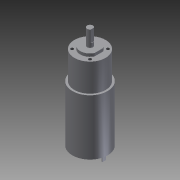
# Autodesk Inventor part: IG32P-Motor
Saved by Autodesk Inventor 2012 (Build 160160000, 160)
## iProperties
Created: 2013-07-13
Part Number: IG32P-Motor
Material: Default
Document SubType Name: Modeling
Designer: joe_000
Density: 2.67636 g/cm^3
Mass: 220 g
Surface Area: 122.703 cm^2
Volume: 82.2012 cm^3
Author: joe_000
Autodesk Inventor part; units mm, degrees
ref_plane "YZ Plane" through (0, 0, 0) normal (1, 0, 0) x (0, 1, 0)
ref_plane "XZ Plane" through (0, 0, 0) normal (0, 1, 0) x (-1, 0, 0)
ref_plane "XY Plane" through (0, 0, 0) normal (0, 0, 1) x (1, 0, 0)
sketch "Sketch1" plane through (0, 0, 0) normal (0, 0, 1) x (1, 0, 0)
  circle A0 centre (0, 0) radius 18
  dimension "d0" = 36
  constraints: 1 centre point, 1 coincident
  measures "d0" diameter of A0
extrude "Extrusion1" add sketch "Sketch1" along normal blind 57.1
sketch "Sketch2" plane through (0, 0, 57.1) normal (0, 0, 1) x (1, 0, 0)
  circle A0 centre (0, 0) radius 16
  dimension "d3" = 32
  constraints: 1 centre point
  measures "d3" diameter of A0
extrude "Extrusion2" add sketch "Sketch2" along normal blind 28.5
sketch "Sketch3" plane through (0, 0, 85.6) normal (0, 0, 1) x (1, 0, 0)
  line L0 (-9, 4.3589) -> (-9, -4.3589)
  line L1 (9, 4.3589) -> (9, -4.3589)
  arc A0 (9, 4.3589) -> (-9, 4.3589) centre (0, 0) ccw
  arc A1 (-9, -4.3589) -> (9, -4.3589) centre (0, 0) ccw
  circle A2 centre (0, 0) radius 16 projected
  dimension "d7" = 18
  dimension "d8" = 9
  dimension "d9" = 10
  dimension "d10" = 10
  constraints: 4 end point, 4 point on circle, 2 centre point, 1 concentric, 1 parallel, 1 vertical
  measures "d7" distance between parallel lines of L1 L0
  measures "d8" distance from line of L1 A0.centre
  measures "d9" radius of A1
  measures "d10" radius of A0
extrude "Extrusion3" add sketch "Sketch3" along normal blind 3 contours A0 L1 A1 L0
sketch "Sketch4" plane through (0, 0, 88.6) normal (0, 0, 1) x (1, 0, 0)
  arc A0 (-9, -4.3589) -> (9, -4.3589) centre (0, 0) ccw projected
  circle A1 centre (0, 0) radius 3
  dimension "d13" = 6
  constraints: 1 centre point, 1 coincident
  measures "d13" diameter of A1
extrude "Extrusion4" add sketch "Sketch4" along normal blind 16.3
sketch "Sketch5" plane through (0, 0, 104.9) normal (0, 0, 1) x (1, 0, 0)
  circle A0 centre (0, 0) radius 3 projected
  line L0 (2.5, 1.6583) -> (2.5, -1.6583)
  dimension "d16" = 2.5
  constraints: 2 end point, 2 point on circle, 1 vertical
  measures "d16" distance from line of A0.centre L0
extrude "Extrusion5" cut sketch "Sketch5" against normal blind 12 contours A0 L0 picked at (2.5914, -0.3806)
sketch "Sketch6" plane through (0, 0, 85.6) normal (0, 0, 1) x (1, 0, 0)
  circle A0 centre (0, 0) radius 16 projected
  circle A1 centre (0, 0) radius 13
  line L0 (0, 0) -> (-9.1924, 9.1924)
  line L1 (0, 0) -> (-13, 0)
  dimension "d19" = 26
  dimension "d20" = 45
  constraints: 4 end point, 2 point on circle, 1 centre point, 1 coincident, 1 horizontal
  measures "d19" diameter of A1
  measures "d20" angle of L0 L1
hole "Hole1" at (-9.1924, 9.1924, 85.6) direction (0, 0, -1) diameter 3 depth 8
pattern_circular "Circular Pattern1" count 4 over 360 about axis through (0, 0, 57.1) along (0, 0, 1) of "Hole1"
thread "Thread1" size "M3x0.5" class "6H" standard "ANSI Metric M Profile" full length
thread "Thread2" size "M3x0.5" class "6H" standard "ANSI Metric M Profile" full length
thread "Thread3" size "M3x0.5" class "6H" standard "ANSI Metric M Profile" full length
thread "Thread4" size "M3x0.5" class "6H" standard "ANSI Metric M Profile" full length
sketch "Sketch7" plane through (0, 0, 0) normal (0, 0, -1) x (-1, 0, 0)
  line L0 (-14.6, 1.91) -> (-14, 1.91)
  line L1 (-14, 1.91) -> (-14, -1.91)
  line L2 (-14, -1.91) -> (-14.6, -1.91)
  line L3 (-14.6, -1.91) -> (-14.6, 1.91)
  line L4 (14, 1.91) -> (14.6, 1.91)
  line L5 (14.6, 1.91) -> (14.6, -1.91)
  line L6 (14.6, -1.91) -> (14, -1.91)
  line L7 (14, -1.91) -> (14, 1.91)
  point P0 (0, 0)
  point P1 (-14, 0)
  point P2 (14, 0)
  dimension "d39" = 3.82
  dimension "d40" = 0.6
  dimension "d41" = 3.82
  dimension "d42" = 0.6
  dimension "d43" = 28
  dimension "d44" = 14
  constraints: 16 end point, 4 parallel, 2 horizontal, 2 midpoint, 2 perpendicular
  measures "d39" distance of L4.end L5.end
  measures "d40" distance of L5.end L6.end
  measures "d41" distance of L2.end L0.start
  measures "d42" distance of L1.end L2.end
  measures "d43" distance between parallel lines of L7 L1
  measures "d44" distance from line of point (0, 0) L1
extrude "Extrusion6" add sketch "Sketch7" along normal blind 6.7
body "Solid1"
